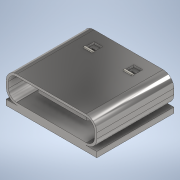
# Autodesk Inventor part: Port 4
Saved by Autodesk Inventor 2020 (Build 240168000, 168)
## iProperties
Created: 2022-11-24
Part Number: Port 4
Material: Generic
Document SubType Name: Modeling
Designer: DELL
Density: 1 g/cm^3
Appearance: Steel - Polished
Author: DELL
Autodesk Inventor part; units mm, degrees
ref_plane "YZ Plane" through (0, 0, 0) normal (1, 0, 0) x (0, 1, 0)
ref_plane "XZ Plane" through (0, 0, 0) normal (0, 1, 0) x (-1, 0, 0)
ref_plane "XY Plane" through (0, 0, 0) normal (0, 0, 1) x (1, 0, 0)
sketch "Sketch1" plane through (0, 0, 0) normal (0, 1, 0) x (-1, 0, 0)
  line L0 (0, 0) -> (0, 14.221)
  line L1 (0, 14.221) -> (-16.746, 14.221)
  line L2 (-16.746, 14.221) -> (-16.746, 0)
  line L3 (-16.746, 0) -> (0, 0)
  dimension "d0" = 14.221
  dimension "d1" = 16.746
  constraints: 8 end point, 3 perpendicular, 1 vertical
  measures "d0" distance of L0.start L0.end
  measures "d1" distance of L0.end L1.end
extrude "Extrusion1" add sketch "Sketch1" along normal blind 6
sketch "Sketch2" plane through (0, 0, 14.221) normal (0, 0, 1) x (1, 0, 0)
  line L0 (16.746, 6) -> (0, 6) projected
  line L1 (2, 6) -> (14.746, 6)
  line L2 (16.746, 4) -> (16.746, 3)
  line L3 (16.746, 0) -> (0, 0) projected
  line L4 (16.746, 0) -> (0, 0)
  line L5 (0, 3) -> (0, 4)
  line L6 (0, 0) -> (0, 6) projected
  line L7 (0, 0) -> (0, 1)
  line L8 (2, 1) -> (14.746, 1)
  line L9 (16.746, 0) -> (16.746, 6) projected
  line L10 (0, 0) -> (16.746, 0)
  line L11 (1.5, 6) -> (0, 6)
  line L12 (0, 6) -> (0, 4.5)
  line L13 (0, 2.5) -> (0, 1)
  line L14 (1.5, 1) -> (0, 1)
  line L15 (15.246, 6) -> (16.746, 6)
  line L16 (16.746, 6) -> (16.746, 4.5)
  line L17 (16.746, 2.5) -> (16.746, 1)
  line L18 (15.246, 1) -> (16.746, 1)
  line L19 (1.9393, 5.5607) -> (14.8067, 5.5607)
  line L20 (16.3067, 4.0607) -> (16.3067, 2.9393)
  line L21 (14.8067, 1.4393) -> (1.9393, 1.4393)
  line L22 (0.4393, 2.9393) -> (0.4393, 4.0607)
  arc A0 (1.9393, 5.5607) -> (0.4393, 4.0607) centre (1.9393, 4.0607) ccw
  arc A1 (16.3067, 4.0607) -> (14.8067, 5.5607) centre (14.8067, 4.0607) ccw
  arc A2 (14.8067, 1.4393) -> (16.3067, 2.9393) centre (14.8067, 2.9393) ccw
  arc A3 (0.4393, 2.9393) -> (1.9393, 1.4393) centre (1.9393, 2.9393) ccw
  line L23 (1.9393, 4.0607) -> (14.8067, 4.0607)
  line L24 (14.8067, 4.0607) -> (14.8067, 2.9393)
  line L25 (14.8067, 2.9393) -> (1.9393, 2.9393)
  line L26 (1.9393, 2.9393) -> (1.9393, 4.0607)
  line L27 (2.409, 4.0607) -> (2.8745, 4.0607)
  line L28 (2.8745, 4.0607) -> (2.8745, 3.8994)
  line L29 (2.8745, 3.8994) -> (2.409, 3.8994)
  line L30 (2.409, 3.8994) -> (2.409, 4.0607)
  line L31 (3.9245, 4.0607) -> (3.9245, 3.8994)
  line L32 (3.459, 4.0607) -> (3.9245, 4.0607)
  line L33 (3.459, 3.8994) -> (3.459, 4.0607)
  line L34 (3.9245, 3.8994) -> (3.459, 3.8994)
  line L35 (4.9745, 4.0607) -> (4.9745, 3.8994)
  line L36 (4.509, 4.0607) -> (4.9745, 4.0607)
  line L37 (4.509, 3.8994) -> (4.509, 4.0607)
  line L38 (4.9745, 3.8994) -> (4.509, 3.8994)
  line L39 (6.0245, 4.0607) -> (6.0245, 3.8994)
  line L40 (5.559, 4.0607) -> (6.0245, 4.0607)
  line L41 (5.559, 3.8994) -> (5.559, 4.0607)
  line L42 (6.0245, 3.8994) -> (5.559, 3.8994)
  line L43 (7.0745, 4.0607) -> (7.0745, 3.8994)
  line L44 (6.609, 4.0607) -> (7.0745, 4.0607)
  line L45 (6.609, 3.8994) -> (6.609, 4.0607)
  line L46 (7.0745, 3.8994) -> (6.609, 3.8994)
  line L47 (8.1245, 4.0607) -> (8.1245, 3.8994)
  line L48 (7.659, 4.0607) -> (8.1245, 4.0607)
  line L49 (7.659, 3.8994) -> (7.659, 4.0607)
  line L50 (8.1245, 3.8994) -> (7.659, 3.8994)
  line L51 (9.1745, 4.0607) -> (9.1745, 3.8994)
  line L52 (8.709, 4.0607) -> (9.1745, 4.0607)
  line L53 (8.709, 3.8994) -> (8.709, 4.0607)
  line L54 (9.1745, 3.8994) -> (8.709, 3.8994)
  line L55 (10.2245, 4.0607) -> (10.2245, 3.8994)
  line L56 (9.759, 4.0607) -> (10.2245, 4.0607)
  line L57 (9.759, 3.8994) -> (9.759, 4.0607)
  line L58 (10.2245, 3.8994) -> (9.759, 3.8994)
  line L59 (11.2745, 4.0607) -> (11.2745, 3.8994)
  line L60 (10.809, 4.0607) -> (11.2745, 4.0607)
  line L61 (10.809, 3.8994) -> (10.809, 4.0607)
  line L62 (11.2745, 3.8994) -> (10.809, 3.8994)
  line L63 (12.3245, 4.0607) -> (12.3245, 3.8994)
  line L64 (11.859, 4.0607) -> (12.3245, 4.0607)
  line L65 (11.859, 3.8994) -> (11.859, 4.0607)
  line L66 (12.3245, 3.8994) -> (11.859, 3.8994)
  line L67 (13.3745, 4.0607) -> (13.3745, 3.8994)
  line L68 (12.909, 4.0607) -> (13.3745, 4.0607)
  line L69 (12.909, 3.8994) -> (12.909, 4.0607)
  line L70 (13.3745, 3.8994) -> (12.909, 3.8994)
  line L71 (14.4245, 4.0607) -> (14.4245, 3.8994)
  line L72 (13.959, 4.0607) -> (14.4245, 4.0607)
  line L73 (13.959, 3.8994) -> (13.959, 4.0607)
  line L74 (14.4245, 3.8994) -> (13.959, 3.8994)
  arc A4 (0, 3) -> (2, 1) centre (2, 3) ccw
  arc A5 (2, 6) -> (0, 4) centre (2, 4) ccw
  arc A6 (16.746, 4) -> (14.746, 6) centre (14.746, 4) ccw
  arc A7 (14.746, 1) -> (16.746, 3) centre (14.746, 3) ccw
  line L75 (1.5, 6) -> (2, 6)
  line L76 (0, 4.5) -> (0, 4)
  line L77 (0, 3) -> (0, 2.5)
  line L78 (1.5, 1) -> (2, 1)
  line L79 (15.246, 1) -> (14.746, 1)
  line L80 (16.746, 2.5) -> (16.746, 3)
  line L81 (16.746, 4) -> (16.746, 4.5)
  line L82 (15.246, 6) -> (14.746, 6)
  line L83 (16.746, 1) -> (16.746, 0)
  point P0 (0.4393, 5.5607)
  point P1 (16.3067, 1.4393)
  dimension "d4" = 1
  dimension "d6" = 1.5
  dimension "d9" = 1.05
  dimension "d14" = 2
  constraints: 158 end point, 44 horizontal alignment, 34 collinear, 27 parallel, 24 point on line, 19 point on circle, 19 tangent, 9 perpendicular, 8 centre point, 6 equal radius, 3 horizontal, 1 midpoint, 1 vertical, 4 other
  measures "d4" distance of L3.end L7.end
  measures "d6" radius of A0
  measures "d9" distance of L27.end L31.start
  measures "d14" radius of A4
extrude "Extrusion2" cut sketch "Sketch2" against normal blind 15 contours L9 A6 L0 | A5 L6 L0 | L9 L18 L79 A7 | A4 L78 L14 L6
extrude "Extrusion3" cut sketch "Sketch2" against normal blind 13 contours L19 A1 L20 A2 L21 A3 L22 A0 | L23 L28 L29 L30 | L23 L31 L34 L33 | L71 L74 L73 L23 | L23 L35 L38 L37 | L67 L70 L69 L23 | L23 L39 L42 L41 | L63 L66 L65 L23 | L23 L43 L46 L45 | L59 L62 L61 L23 | L23 L47 L50 L49 | L55 L58 L57 L23 | L23 L51 L54 L53
extrude "Extrusion4" add sketch "Sketch2" against normal blind 2 contours L23 L30 L29 L28 L33 L34 L31 L37 L38 L35 L41 L42 L39 L45 L46 L43 L49 L50 L47 L53 L54 L51 L57 L58 L55 L61 L62 L59 L65 L66 L63 L69 L70 L67 L73 L74 L71 L24 L25 L26
extrude "Extrusion5" cut sketch "Sketch2" against normal blind 2 contours L23 L30 L29 L28 L33 L34 L31 L37 L38 L35 L41 L42 L39 L45 L46 L43 L49 L50 L47 L53 L54 L51 L57 L58 L55 L61 L62 L59 L65 L66 L63 L69 L70 L67 L73 L74 L71 L24 L25 L26
chamfer "Chamfer1" distance 2 angle 45 1 edges at (14.8067, 3.5, 12.221)
chamfer "Chamfer2" distance 2 angle 45 1 edges at (1.9393, 3.5, 12.221)
sketch "Sketch3" plane through (0, 6, 0) normal (0, 1, 0) x (1, 0, 0)
  line L0 (3.9245, -12.2062) -> (3.9245, -1.221) projected
  line L1 (3.9245, -1.9149) -> (3.9245, -3.3149)
  line L2 (3.9245, -3.3149) -> (5.5245, -3.3149)
  line L3 (3.9245, -1.9149) -> (5.5245, -1.9149)
  line L4 (5.5245, -1.9149) -> (5.5245, -3.3149)
  line L5 (5.559, -12.221) -> (5.559, -1.221) projected
  line L6 (12.909, -12.1187) -> (12.909, -1.221) projected
  line L7 (12.909, -3.3149) -> (12.909, -1.9149)
  line L8 (12.909, -1.9149) -> (11.2745, -1.9149)
  line L9 (11.2745, -12.221) -> (11.2745, -1.221) projected
  line L10 (11.2745, -3.3149) -> (11.2745, -1.9149)
  line L11 (11.2745, -3.3149) -> (12.909, -3.3149)
  point P0 (0, 0)
  point P1 (5.559, -1.221)
  dimension "d29" = 1.4
  dimension "d30" = 1.6
  constraints: 16 end point, 5 point on line, 3 perpendicular, 2 vertical, 1 collinear, 1 horizontal, 1 other
  measures "d29" distance of L1.start L1.end
  measures "d30" distance of L1.end L2.end
extrude "Extrusion6" cut sketch "Sketch3" against normal blind 0.7
sketch "Sketch4" plane through (0, 6, 0) normal (0, 1, 0) x (1, 0, 0)
  line L0 (3.9245, -3.8908) -> (3.9245, -3.3149)
  line L1 (11.2745, -3.3149) -> (12.909, -3.3149) projected
  line L2 (11.2745, -3.8908) -> (11.2745, -3.3149)
  line L3 (11.2745, -3.3149) -> (12.909, -3.3149)
  line L4 (12.909, -12.1187) -> (12.909, -1.221) projected
  line L5 (12.909, -3.8908) -> (11.2745, -3.8908)
  line L6 (12.909, -3.3149) -> (12.909, -3.8908)
  line L7 (3.9245, -3.3149) -> (5.559, -3.3149)
  line L8 (3.9245, -3.8908) -> (5.559, -3.8908)
  line L9 (5.559, -12.221) -> (5.559, -1.221) projected
  line L10 (5.559, -3.3149) -> (5.559, -3.8908)
  point P0 (0, 0)
  constraints: 16 end point, 2 collinear, 2 horizontal, 2 perpendicular, 2 point on line
extrude "Extrusion7" add sketch "Sketch4" along normal blind 0.2
chamfer "Chamfer3" distance 0.25 angle 45 2 edges at (4.7417, 6.2, 3.3149) (12.0917, 6.2, 3.3149)
body "Solid1"
